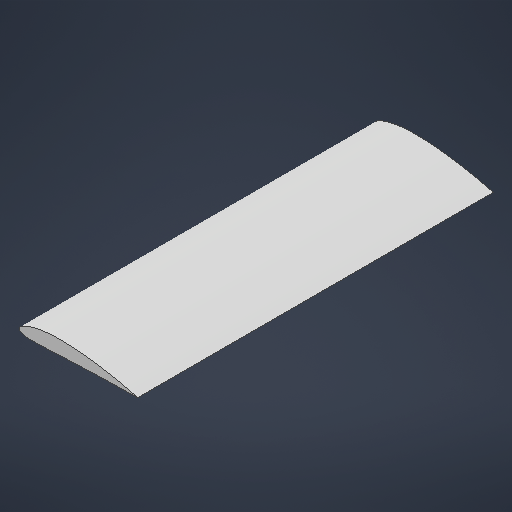
# Autodesk Inventor part: Part1
Saved by Autodesk Inventor 2026 (Build 300175050, 175E)
## iProperties
Created: 2025-05-27
Part Number: Part1
Material: Generic
Document SubType Name: Modeling
Designer: deniatmojoo
Density: 1 g/cm^3
Appearance: Default
Author: deniatmojoo
Autodesk Inventor part; units mm, degrees
ref_plane "YZ Plane" through (0, 0, 0) normal (1, 0, 0) x (0, 1, 0)
ref_plane "XZ Plane" through (0, 0, 0) normal (0, 1, 0) x (-1, 0, 0)
ref_plane "XY Plane" through (0, 0, 0) normal (0, 0, 1) x (1, 0, 0)
sketch "Sketch1" plane through (0, 0, 0) normal (0, 0, 1) x (1, 0, 0)
  line L0 (0, 0) -> (1.25, 2.44) construction
  line L1 (1.25, 2.44) -> (2.5, 3.39) construction
  line L2 (2.5, 3.39) -> (5, 4.73) construction
  line L3 (5, 4.73) -> (7.5, 5.76) construction
  line L4 (7.5, 5.76) -> (10, 6.59) construction
  line L5 (10, 6.59) -> (15, 7.89) construction
  line L6 (15, 7.89) -> (20, 8.8) construction
  line L7 (20, 8.8) -> (25, 9.41) construction
  line L8 (25, 9.41) -> (30, 9.76) construction
  line L9 (30, 9.76) -> (40, 9.76) construction
  line L10 (40, 9.76) -> (50, 9.19) construction
  line L11 (50, 9.19) -> (60, 8.14) construction
  line L12 (60, 8.14) -> (70, 6.69) construction
  line L13 (70, 6.69) -> (80, 4.89) construction
  line L14 (80, 4.89) -> (90, 2.71) construction
  line L15 (90, 2.71) -> (95, 1.47) construction
  line L16 (95, 1.47) -> (100, 0.13) construction
  line L17 (100, 0.13) -> (100.4093, 0) construction
  spline S0 degree 4 poles (0, 0) (1.25, 2.44) (2.5, 3.39) (5, 4.73) (7.5, 5.76) (10, 6.59) (15, 7.89) (20, 8.8) (25, 9.41) (30, 9.76) (40, 9.76) (50, 9.19) (60, 8.14) (70, 6.69) (80, 4.89) (90, 2.71) (95, 1.47) (100, 0.13) (100.4093, 0) knots 1 1 1 1 1 2 3 4 5 6 7 8 9 10 11 12 13 14 15 16 16 16 16 16
  line L18 (0, 0) -> (1.25, -1.43) construction
  line L19 (1.25, -1.43) -> (2.5, -1.95) construction
  line L20 (2.5, -1.95) -> (4.9968, -2.4943) construction
  line L21 (4.9968, -2.4943) -> (7.4982, -2.757) construction
  line L22 (7.4982, -2.757) -> (9.9978, -2.8994) construction
  line L23 (9.9978, -2.8994) -> (15, -2.8994) construction
  line L24 (15, -2.8994) -> (20, -2.74) construction
  line L25 (20, -2.74) -> (25, -2.5) construction
  line L26 (25, -2.5) -> (30, -2.26) construction
  line L27 (30, -2.26) -> (40, -1.8) construction
  line L28 (40, -1.8) -> (50, -1.4) construction
  line L29 (50, -1.4) -> (60, -1) construction
  line L30 (60, -1) -> (70, -0.65) construction
  line L31 (70, -0.65) -> (80, -0.39) construction
  line L32 (80, -0.39) -> (90, -0.22) construction
  line L33 (90, -0.22) -> (95, -0.16) construction
  line L34 (95, -0.16) -> (100, -0.13) construction
  line L35 (100, -0.13) -> (100.4093, 0) construction
  spline S1 degree 4 poles (0, 0) (1.25, -1.43) (2.5, -1.95) (4.9968, -2.4943) (7.4982, -2.757) (9.9978, -2.8994) (15, -2.8994) (20, -2.74) (25, -2.5) (30, -2.26) (40, -1.8) (50, -1.4) (60, -1) (70, -0.65) (80, -0.39) (90, -0.22) (95, -0.16) (100, -0.13) (100.4093, 0) knots 1 1 1 1 1 2 3 4 5 6 7 8 9 10 11 12 13 14 15 16 16 16 16 16
  point P0 (5, 4.73)
  point P1 (30, -2.26)
  constraints: 34 coincident, 2 horizontal, 6 other
extrude "Extrusion1" add sketch "Sketch1" along normal mid plane 300
body "Solid1"
